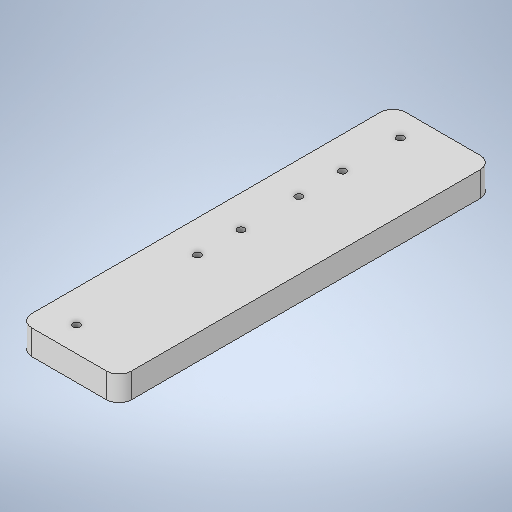
# Autodesk Inventor part: Base barramentos
Saved by Autodesk Inventor 2025 (Build 290162000, 162)
## iProperties
Created: 2024-09-28
Part Number: Base barramentos
Material: Genérico
Document SubType Name: Modeling
Designer: phmca
Density: 1 g/cm^3
Appearance: Padrão
Author: phmca
Autodesk Inventor part; units mm, degrees
ref_plane "YZ Plane" through (0, 0, 0) normal (1, 0, 0) x (0, 1, 0)
ref_plane "XZ Plane" through (0, 0, 0) normal (0, 1, 0) x (-1, 0, 0)
ref_plane "XY Plane" through (0, 0, 0) normal (0, 0, 1) x (1, 0, 0)
sketch "Esboço1" plane through (0, 0, 0) normal (0, 1, 0) x (-1, 0, 0)
  line L0 (20, 75) -> (-20, 75)
  line L1 (-20, 75) -> (-20, -75)
  line L2 (-20, -75) -> (20, -75)
  line L3 (20, -75) -> (20, 75)
  line L4 (7.1, 63.25) -> (7.1, 18.19) construction
  circle A0 centre (7.1, 16.44) radius 1.75 construction
  circle A1 centre (7.1, 65) radius 1.75 construction
  line L5 (7.1, 65) -> (7.1, 63.25) construction
  line L6 (7.1, 16.44) -> (7.1, 18.19) construction
  circle A2 centre (7.1, 16.44) radius 1.45
  circle A3 centre (7.1, 65) radius 1.45
  line L7 (14.5, 62.22) -> (-14.5, 62.22) construction
  line L8 (-14.5, 62.22) -> (-14.5, 19.22) construction
  line L9 (-14.5, 19.22) -> (14.5, 19.22) construction
  line L10 (14.5, 19.22) -> (14.5, 62.22) construction
  line L11 (11.1, 61) -> (3.1, 61) construction
  line L12 (3.1, 61) -> (3.1, 69) construction
  line L13 (3.1, 69) -> (11.1, 69) construction
  line L14 (11.1, 69) -> (11.1, 61) construction
  line L15 (11.1, 61) -> (3.1, 69) construction
  line L16 (3.1, 61) -> (11.1, 69) construction
  line L17 (3.1, 20.44) -> (11.1, 20.44) construction
  line L18 (11.1, 20.44) -> (11.1, 12.44) construction
  line L19 (11.1, 12.44) -> (3.1, 12.44) construction
  line L20 (3.1, 12.44) -> (3.1, 20.44) construction
  line L21 (3.1, 20.44) -> (11.1, 12.44) construction
  line L22 (11.1, 20.44) -> (3.1, 12.44) construction
  line L23 (7.1, 40.72) -> (7.6918, 40.72) construction
  line L24 (14.5, 40.72) -> (22.5062, 40.72) construction
  line L25 (7.1, -1.12) -> (7.1, -24.28) construction
  circle A4 centre (7.1, -1.12) radius 1.45
  circle A5 centre (7.1, -24.28) radius 1.45
  circle A6 centre (7.1, -41.84) radius 1.45
  circle A7 centre (7.1, -65) radius 1.45
  line L26 (7.1, -41.84) -> (7.1, -65) construction
  line L27 (7.1, 16.44) -> (7.1, -1.12) construction
  line L28 (7.1, -24.28) -> (7.1, -41.84) construction
  line L29 (0, 62.22) -> (0, 19.22) construction
  line L30 (0, 75) -> (0, 85.6082) construction
  point P0 (0, 0)
  dimension "d5" = 3.5
  dimension "d6" = 3.5
  dimension "d0" = 150
  dimension "d1" = 40
  dimension "d2" = 20
  dimension "d3" = 75
  dimension "d4" = 45.06
  dimension "d7" = 2.9
  dimension "d8" = 2.9
  dimension "d9" = 48.56
  dimension "d10" = 29
  dimension "d11" = 8
  dimension "d12" = 8
  dimension "d13" = 8
  dimension "d14" = 8
  dimension "d15" = 3.4
  dimension "d16" = 43
  dimension "d17" = 2.9
  dimension "d18" = 2.9
  dimension "d19" = 23.16
  dimension "d20" = 2.9
  dimension "d21" = 2.9
  dimension "d22" = 23.16
  dimension "d23" = 10
  dimension "d24" = 10
  constraints: 62 end point, 9 midpoint, 8 parallel, 7 vertical, 6 centre point, 6 collinear, 6 perpendicular, 5 horizontal, 4 coincident, 2 vertical alignment, 4 other
  measures "d0" distance of L2.end L0.start
  measures "d1" distance of L1.end L2.end
  measures "d2" horizontal distance of L2.end point (0, 0)
  measures "d3" distance from line of L0 point (0, 0)
  measures "d4" distance of L4.start L4.end
  measures "d7" diameter of A2
  measures "d8" diameter of A3
  measures "d9" distance of L6.start L5.start
  measures "d10" distance of L8.end L9.end
  measures "d11" distance of L12.end L13.end
  measures "d12" distance of L11.end L12.end
  measures "d13" distance of L19.end L17.start
  measures "d14" distance of L18.end L19.end
  measures "d15" distance between parallel lines of L10 L14
  measures "d16" distance of L7.end L8.end
  measures "d17" diameter of A4
  measures "d18" diameter of A5
  measures "d19" distance of L25.start L25.end
  measures "d20" diameter of A6
  measures "d21" diameter of A7
  measures "d22" distance of L26.end L26.start
  measures "d23" distance from line of L0 L5.start
  measures "d24" distance from line of L2 L26.end
extrude "Extrusão1" add sketch "Esboço1" along normal blind 10 contours L3 L2 L1 L0 | A2 | A3 | A4 | A5 | A6 | A7
sketch "Esboço2" plane through (0, 10, 0) normal (0, 1, 0) x (1, 0, 0)
  circle A0 centre (-7.1, -65) radius 1.45 projected
  circle A1 centre (-7.1, -16.44) radius 1.45 projected
  circle A2 centre (-7.1, 1.12) radius 1.45 projected
  circle A3 centre (-7.1, 24.28) radius 1.45 projected
  circle A4 centre (-7.1, 41.84) radius 1.45 projected
  circle A5 centre (-7.1, 65) radius 1.45 projected
  point P0 (0, 0)
extrude "Extrusão2" cut sketch "Esboço2" against normal blind 8.5
fillet "Arredondamento1" radius 5 4 edges at (20, 5, 75) (-20, 5, 75) (20, 5, -75) (-20, 5, -75)
equation "\"d2\" = 0.5 * d1"
equation "\"d3\" = 0.5 * d0"
equation "\"d12\" = d11"
equation "\"d13\" = d12"
equation "\"d14\" = d12"
equation "\"d17\" = d8"
equation "\"d18\" = d17"
equation "\"d20\" = d18"
equation "\"d21\" = d18"
equation "\"d22\" = d19"
equation "\"d24\" = d23"
